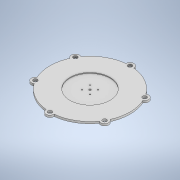
# Autodesk Inventor part: Base
Saved by Autodesk Inventor 2022 (Build 260153000, 153)
## iProperties
Created: 2022-01-07
Part Number: Base
Material: Generic
Document SubType Name: Modeling
Designer: nguye
Density: 1 g/cm^3
Appearance: Default
Author: nguye
Autodesk Inventor part; units mm, degrees
ref_plane "YZ Plane" through (0, 0, 0) normal (1, 0, 0) x (0, 1, 0)
ref_plane "XZ Plane" through (0, 0, 0) normal (0, 1, 0) x (-1, 0, 0)
ref_plane "XY Plane" through (0, 0, 0) normal (0, 0, 1) x (1, 0, 0)
sketch "Sketch1" plane through (0, 0, 0) normal (0, 1, 0) x (-1, 0, 0)
  arc A0 (9.9875, 99.5) -> (-9.9875, 99.5) centre (0, 100) ccw
  arc A1 (91.1633, 41.1006) -> (81.1758, 58.3994) centre (86.6025, 50) ccw
  arc A2 (81.1758, -58.3994) -> (91.1633, -41.1006) centre (86.6025, -50) ccw
  arc A3 (-9.9875, -99.5) -> (9.9875, -99.5) centre (0, -100) ccw
  arc A4 (-91.1633, -41.1006) -> (-81.1758, -58.3994) centre (-86.6025, -50) ccw
  arc A5 (-81.1758, 58.3994) -> (-91.1633, 41.1006) centre (-86.6025, 50) ccw
  arc A6 (81.1758, 58.3994) -> (9.9875, 99.5) centre (0, 0) ccw
  arc A7 (91.1633, -41.1006) -> (91.1633, 41.1006) centre (0, 0) ccw
  arc A8 (9.9875, -99.5) -> (81.1758, -58.3994) centre (0, 0) ccw
  arc A9 (-81.1758, -58.3994) -> (-9.9875, -99.5) centre (0, 0) ccw
  arc A10 (-9.9875, 99.5) -> (-81.1758, 58.3994) centre (0, 0) ccw
  arc A11 (-91.1633, 41.1006) -> (-91.1633, -41.1006) centre (0, 0) ccw
  circle A12 centre (0, 100) radius 5
  circle A13 centre (86.6025, 50) radius 5
  circle A14 centre (86.6025, -50) radius 5
  circle A15 centre (0, -100) radius 5
  circle A16 centre (-86.6025, -50) radius 5
  circle A17 centre (-86.6025, 50) radius 5
  dimension "d3" = 20
  dimension "d4" = 20
  dimension "d5" = 20
  dimension "d6" = 20
  dimension "d7" = 20
  dimension "d8" = 20
  dimension "d9" = 10
  dimension "d10" = 10
  dimension "d11" = 10
  dimension "d12" = 10
  dimension "d13" = 10
  dimension "d14" = 10
  constraints: 24 point on circle, 18 centre point, 7 coincident
  measures "d3" diameter of A0
  measures "d4" diameter of A1
  measures "d5" diameter of A2
  measures "d6" diameter of A3
  measures "d7" diameter of A4
  measures "d8" diameter of A5
  measures "d9" diameter of A12
  measures "d10" diameter of A13
  measures "d11" diameter of A14
  measures "d12" diameter of A15
  measures "d13" diameter of A16
  measures "d14" diameter of A17
extrude "Extrusion1" add sketch "Sketch1" along normal blind 5
sketch "Sketch2" plane through (0, 5, 0) normal (0, 1, 0) x (1, 0, 0)
  circle A0 centre (0, 0) radius 50
  dimension "d17" = 100
  constraints: 1 centre point, 1 coincident
  measures "d17" diameter of A0
extrude "Extrusion2" cut sketch "Sketch2" against normal blind 2
sketch "Sketch3" plane through (0, 3, 0) normal (0, 1, 0) x (1, 0, 0)
  circle A0 centre (0, 0) radius 2.5
  circle A1 centre (-10, -10) radius 1.5
  circle A2 centre (-10, 10) radius 1.5
  circle A3 centre (10, 10) radius 1.5
  circle A4 centre (10, -10) radius 1.5
  dimension "d20" = 5
  dimension "d29" = 3
  dimension "d30" = 3
  dimension "d31" = 3
  dimension "d32" = 3
  constraints: 5 centre point, 1 coincident
  measures "d20" diameter of A0
  measures "d29" diameter of A1
  measures "d30" diameter of A2
  measures "d31" diameter of A3
  measures "d32" diameter of A4
extrude "Extrusion3" cut sketch "Sketch3" against normal blind 5
body "Solid1"
